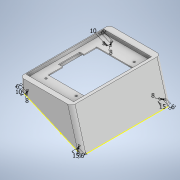
# Autodesk Inventor part: Front
Saved by Autodesk Inventor 2022 (Build 260153000, 153)
## iProperties
Created: 2021-06-27
Part Number: Front
Material: Generic
Document SubType Name: Modeling
Designer: Anton
Density: 1 g/cm^3
Appearance: Default
Author: Anton
Autodesk Inventor part; units mm, degrees
ref_plane "YZ Plane" through (0, 0, 0) normal (1, 0, 0) x (0, 1, 0)
ref_plane "XZ Plane" through (0, 0, 0) normal (0, 1, 0) x (-1, 0, 0)
ref_plane "XY Plane" through (0, 0, 0) normal (0, 0, 1) x (1, 0, 0)
sketch "Sketch1" plane through (0, 0, 0) normal (0, 1, 0) x (-1, 0, 0)
  line L0 (8, 0) -> (102.94, 0)
  line L1 (110.94, -8) -> (110.94, -185.2)
  line L2 (102.94, -193.2) -> (8, -193.2)
  line L3 (0, -185.2) -> (0, -8)
  circle A0 centre (86.7029, -32) radius 2.1
  circle A1 centre (88.297, -158.2) radius 2.1
  circle A2 centre (22.6, -158.501) radius 2.1
  circle A3 centre (21.4029, -32) radius 2.1
  arc A4 (110.94, -8) -> (102.94, 0) centre (102.94, -8) ccw
  arc A5 (8, 0) -> (0, -8) centre (8, -8) ccw
  arc A6 (0, -185.2) -> (8, -193.2) centre (8, -185.2) ccw
  arc A7 (102.94, -193.2) -> (110.94, -185.2) centre (102.94, -185.2) ccw
  point P0 (0, 0)
  dimension "d0" = 110.94
  dimension "d1" = 193.2
  dimension "d2" = 4.2
  dimension "d3" = 4.2
  dimension "d4" = 65.3
  dimension "d5" = 65.697
  dimension "d6" = 4.2
  dimension "d7" = 4.2
  dimension "d8" = 126.2
  dimension "d9" = 126.501
  dimension "d10" = 0
  dimension "d11" = 22.6
  dimension "d12" = 35
  dimension "d13" = 8
  constraints: 8 centre point, 8 end point, 8 point on circle, 8 tangent, 3 equal radius, 2 parallel, 2 point on line, 1 horizontal, 1 perpendicular
  measures "d0" distance between parallel lines of L3 L1
  measures "d1" distance between parallel lines of L2 L0
  measures "d2" diameter of A0
  measures "d3" diameter of A3
  measures "d4" distance of A3.centre A0.centre
  measures "d5" horizontal distance of A2.centre A1.centre
  measures "d6" diameter of A1
  measures "d7" diameter of A2
  measures "d8" vertical distance of A1.centre A0.centre
  measures "d9" vertical distance of A2.centre A3.centre
  measures "d10" vertical distance of A0.centre A3.centre
  measures "d11" distance from line of L3 A2.centre
  measures "d12" distance from line of L2 A1.centre
  measures "d13" radius of A4
extrude "Extrusion1" add sketch "Sketch1" along normal blind 2
sketch "Sketch2" plane through (0, 2, 0) normal (0, 1, 0) x (1, 0, 0)
  line L0 (-8, 193.2) -> (-102.94, 193.2) projected
  arc A0 (-102.94, 193.2) -> (-110.94, 185.2) centre (-102.94, 185.2) ccw projected
  line L1 (-110.94, 185.2) -> (-110.94, 8) projected
  arc A1 (-110.94, 8) -> (-102.94, 0) centre (-102.94, 8) ccw projected
  line L2 (-102.94, 0) -> (-8, 0) projected
  arc A2 (-8, 0) -> (0, 8) centre (-8, 8) ccw projected
  line L3 (0, 8) -> (0, 185.2) projected
  arc A3 (0, 185.2) -> (-8, 193.2) centre (-8, 185.2) ccw projected
  circle A4 centre (-86.7029, 32) radius 2.1 projected
  circle A5 centre (-88.297, 158.2) radius 2.1 projected
  circle A6 centre (-22.6, 158.501) radius 2.1 projected
  circle A7 centre (-21.4029, 32) radius 2.1 projected
  line L4 (-108.94, 11) -> (-108.94, 179.2)
  line L5 (-108.94, 179.2) -> (-6, 179.2)
  line L6 (-6, 11) -> (-108.94, 11)
  line L7 (-6, 179.2) -> (-6, 11)
  point P0 (0, 0)
  dimension "d16" = 2
  dimension "d17" = 14
  dimension "d18" = 11
  dimension "d19" = 6
  constraints: 8 end point, 1 horizontal
  measures "d16" distance between parallel lines of L1 L4
  measures "d17" distance between parallel lines of L0 L5
  measures "d18" distance between parallel lines of L2 L6
  measures "d19" distance between parallel lines of L3 L7
extrude "Extrusion2" add sketch "Sketch2" along normal blind 7.5 contours A3 L3 A2 L2 A1 L1 A0 L0
sketch "Sketch3" plane through (0, 2, 0) normal (0, 1, 0) x (1, 0, 0)
  line L0 (-91, 41) -> (-12, 41)
  line L1 (-12, 41) -> (-12, 146)
  line L2 (-12, 146) -> (-91, 146)
  line L3 (-6, 179.2) -> (-6, 11) projected
  line L4 (-6, 11) -> (-108.94, 11) projected
  line L5 (-99.94, 72) -> (-91, 72)
  line L6 (-91, 118.2) -> (-99.94, 118.2)
  line L7 (-99.94, 118.2) -> (-99.94, 72)
  circle A0 centre (-88.297, 158.2) radius 2.1 projected
  circle A1 centre (-86.7029, 32) radius 2.1 projected
  line L8 (-108.94, 11) -> (-108.94, 179.2) projected
  line L9 (-91, 146) -> (-91, 118.2)
  line L10 (-91, 72) -> (-91, 41)
  point P0 (0, 0)
  dimension "d22" = 105
  dimension "d24" = 6
  dimension "d25" = 30
  dimension "d26" = 40
  dimension "d27" = 40
  dimension "d28" = 9
  constraints: 16 end point, 4 parallel, 2 horizontal, 1 perpendicular
  measures "d22" distance between parallel lines of L2 L0
  measures "d24" distance between parallel lines of L3 L1
  measures "d25" distance between parallel lines of L4 L0
  measures "d26" distance from line of L6 A0.centre
  measures "d27" distance from line of L5 A1.centre
  measures "d28" distance between parallel lines of L8 L7
extrude "Extrusion3" cut sketch "Sketch3" against normal blind 7.5 contours L10 L5 L7 L6 L9 L2 L1 L0
sketch "Sketch5" plane through (0, 0, 0) normal (0, -1, 0) x (1, 0, 0)
  line L0 (-12, -146) -> (-91, -146) projected
  line L1 (-91, -146) -> (-91, -118.2) projected
  line L2 (-91, -118.2) -> (-99.94, -118.2) projected
  line L3 (-99.94, -118.2) -> (-99.94, -72) projected
  line L4 (-99.94, -72) -> (-91, -72) projected
  line L5 (-91, -72) -> (-91, -41) projected
  line L6 (-91, -41) -> (-12, -41) projected
  line L7 (-12, -41) -> (-12, -146) projected
  line L8 (-8, -193.2) -> (-102.94, -193.2) projected
  arc A0 (-8, -193.2) -> (0, -185.2) centre (-8, -185.2) ccw projected
  line L9 (0, -8) -> (0, -185.2) projected
  arc A1 (0, -8) -> (-8, 0) centre (-8, -8) ccw projected
  line L10 (-102.94, 0) -> (-8, 0) projected
  arc A2 (-102.94, 0) -> (-110.94, -8) centre (-102.94, -8) ccw projected
  line L11 (-110.94, -185.2) -> (-110.94, -8) projected
  arc A3 (-110.94, -185.2) -> (-102.94, -193.2) centre (-102.94, -185.2) ccw projected
  circle A4 centre (-86.7029, -32) radius 2.1 projected
  circle A5 centre (-88.297, -158.2) radius 2.1 projected
  circle A6 centre (-22.6, -158.501) radius 2.1 projected
  circle A7 centre (-21.4029, -32) radius 2.1 projected
  line L12 (-102.94, -191.2) -> (-8, -191.2)
  arc A8 (-8, -191.2) -> (-2, -185.2) centre (-8, -185.2) ccw
  line L13 (-2, -185.2) -> (-2, -8)
  arc A9 (-2, -8) -> (-8, -2) centre (-8, -8) ccw
  line L14 (-8, -2) -> (-102.94, -2)
  arc A10 (-102.94, -2) -> (-108.94, -8) centre (-102.94, -8) ccw
  line L15 (-108.94, -8) -> (-108.94, -185.2)
  arc A11 (-108.94, -185.2) -> (-102.94, -191.2) centre (-102.94, -185.2) ccw
  point P0 (0, 0)
  dimension "d39" = 2
  constraints: 8 end point, 8 point on circle, 4 centre point, 7 other
  measures "d39" radial gap between concentric circles of A3 A11
extrude "Extrusion4" add sketch "Sketch5" along normal blind 72 contours L8 A3 L11 A2 L10 A1 L9 A0
sketch "Sketch6" plane through (-8, 9.5, -193.2) normal (0, 0, -1) x (-1, 0, 0)
  line L0 (102.94, -81.5) -> (102.94, 0) projected
  line L1 (-8, -81.5) -> (102.94, -81.5)
  line L2 (102.94, -81.5) -> (102.94, -23.5)
  line L3 (102.94, 0) -> (94.94, 0) projected
  line L4 (-8, -81.5) -> (0, -81.5) projected
  line L5 (0, 0) -> (-8, 0) projected
  line L6 (0, 0) -> (94.94, 0) projected
  line L7 (102.94, -23.5) -> (-25.549, -79.0929)
  line L8 (-8, -81.5) -> (-29.8984, -81.5)
  line L9 (-29.8984, -81.5) -> (-31.1125, -81.5)
  line L10 (-25.549, -79.0929) -> (-31.1125, -81.5)
  line L11 (-8, -81.5) -> (-8, 0) projected
  point P0 (-8, -9.5)
  dimension "d42" = 23.5
  dimension "d47" = 23.396
  dimension "d48" = 140
  dimension "d51" = 23.1125
  constraints: 12 end point, 3 horizontal, 1 point on line
  measures "d42" distance from line of L3 L2.end
  measures "d47" angle of L6 L7
  measures "d48" distance of L2.end L7.end
  measures "d51" distance from line of L9.end L11
extrude "Extrusion5" cut sketch "Sketch6" along normal mid plane 1000 contours L1 L11 L7 L0 | L11 L8 L9 L10 L7
sketch "Sketch7" plane through (0, 9.5, 0) normal (0, 1, 0) x (1, 0, 0)
  arc A0 (-102.94, 193.2) -> (-110.94, 185.2) centre (-102.94, 185.2) ccw projected
  line L0 (-110.94, 185.2) -> (-110.94, 8) projected
  arc A1 (-110.94, 8) -> (-102.94, 0) centre (-102.94, 8) ccw projected
  line L1 (-102.94, 0) -> (-8, 0) projected
  arc A2 (-8, 0) -> (0, 8) centre (-8, 8) ccw projected
  line L2 (0, 8) -> (0, 185.2) projected
  arc A3 (0, 185.2) -> (-8, 193.2) centre (-8, 185.2) ccw projected
  line L3 (-8, 193.2) -> (-102.94, 193.2) projected
  line L4 (-108.94, 11) -> (-108.94, 179.2) projected
  line L5 (-108.94, 179.2) -> (-6, 179.2) projected
  line L6 (-6, 179.2) -> (-6, 11) projected
  line L7 (-6, 11) -> (-108.94, 11) projected
  line L8 (-8, 0) -> (23.113, 0)
  arc A4 (-8, 0) -> (0, 8) centre (-8, 8) ccw projected
  line L9 (23.113, 0) -> (23.113, 193.2)
  line L10 (23.113, 193.2) -> (-8, 193.2)
  arc A5 (0, 185.2) -> (-8, 193.2) centre (-8, 185.2) ccw projected
  point P0 (0, 0)
  point P1 (-8, 193.2)
  dimension "d52" = 23.113
  constraints: 6 end point, 2 perpendicular, 2 point on circle, 2 tangent, 1 horizontal
  measures "d52" distance between parallel lines of L2 L9
extrude "Extrusion6" add sketch "Sketch7" against normal up to surface contours L10 L9 L8 A2 L2 A3 surface through (-110.94, -14, -193.2) normal (0.397092, 0.9177788, 0)
sketch "Sketch8" plane through (-102.94, -17.4613, 0) normal (0, 0, 1) x (1, 0, 0)
  line L0 (126.053, 26.9613) -> (0, 26.9613) projected
  line L1 (126.053, 26.9613) -> (102.94, 26.9613)
  line L2 (0, 0) -> (126.053, -54.5389) projected
  line L3 (102.94, 26.9613) -> (126.053, -54.5389)
  line L4 (126.053, 26.9613) -> (126.053, -54.5389) projected
  line L5 (126.053, -54.5389) -> (126.053, 26.9613)
  point P0 (102.94, 17.4613)
  point P1 (96.94, 26.9613)
  dimension "d55" = 6
  constraints: 6 end point, 1 collinear, 1 point on line
  measures "d55" distance of point (96.94, 26.961) L1.end
extrude "Extrusion7" cut sketch "Sketch8" against normal blind 1000
sketch "Sketch9" plane through (0, 9.5, 0) normal (0, 1, 0) x (1, 0, 0)
  line L0 (23.113, 0) -> (0, 0) projected
  line L1 (-8, 0) -> (-110.94, 0)
  line L2 (-110.94, 0) -> (-110.94, 193.2)
  line L3 (-110.94, 193.2) -> (-8, 193.2)
  line L4 (0, 185.2) -> (0, 8)
  arc A0 (0, 185.2) -> (-8, 193.2) centre (-8, 185.2) ccw
  arc A1 (-8, 0) -> (0, 8) centre (-8, 8) ccw
  line L5 (0, 0) -> (0, 193.2) projected
  line L6 (0, 193.2) -> (0, 185.2)
  line L7 (-8, 193.2) -> (0, 193.2)
  line L8 (-102.94, 193.2) -> (23.113, 193.2) projected
  line L9 (-8, 0) -> (0, 0)
  line L10 (23.113, 0) -> (-102.94, 0) projected
  line L11 (0, 8) -> (0, 0)
  dimension "d58" = 8
  constraints: 16 end point, 6 tangent, 5 point on circle, 3 point on line, 2 centre point, 2 collinear, 2 parallel, 2 perpendicular, 1 equal radius, 1 horizontal
  measures "d58" radius of A0
sketch3d "3D Sketch1"
  line L0 (0, 9.5, 0) -> (23.113, -72.0002, 0)
sweep "Sweep1" cut profiles "Sketch9" path "3D Sketch1" contours A1 L5 L9 | A0 L7 L5
ref_plane "Work Plane1" through (23.113, -72.0002, -144.9) normal (-0.272835, 0.9620608, 0) x (0, 0, 1)
sketch "Sketch11" plane through (23.113, -72.0002, -144.9) normal (-0.272835, 0.9620608, 0) x (0, 0, 1)
  line L0 (-46.3, -106.3905) -> (-46.3, -26.2598) projected
  ellipse E0 centre (-40.3, -106.3905) end of major axis (-34.3, -106.3905) minor radius 5.0641 (-46.3, -106.3905) -> (-40.3, -111.4546) ccw projected
  line L1 (136.9, -111.4546) -> (-40.3, -111.4546) projected
  ellipse E1 centre (136.9, -106.3905) end of major axis (142.9, -106.3905) minor radius 5.0641 (136.9, -111.4546) -> (142.9, -106.3905) ccw projected
  line L2 (142.9, -26.2598) -> (142.9, -106.3905) projected
  ellipse E2 centre (136.9, -26.2598) end of major axis (130.9, -26.2598) minor radius 5.0641 (142.9, -26.2598) -> (136.9, -21.1957) ccw projected
  line L3 (-40.3, -21.1957) -> (136.9, -21.1957) projected
  ellipse E3 centre (-40.3, -26.2598) end of major axis (-46.3, -26.2598) minor radius 5.0641 (-40.3, -21.1957) -> (-46.3, -26.2598) ccw projected
  ellipse E4 centre (-40.3, -7.6965) end of major axis (-48.3, -7.6965) minor radius 7.6965 (-40.3, 0) -> (-48.3, -7.6965) ccw projected
  line L4 (-40.3, 0) -> (136.9, 0) projected
  ellipse E5 centre (136.9, -7.6965) end of major axis (144.9, -7.6965) minor radius 7.6965 (144.9, -7.6965) -> (136.9, 0) ccw projected
  line L5 (144.9, -7.6965) -> (144.9, -106.3905) projected
  ellipse E6 centre (136.9, -106.3905) end of major axis (144.9, -106.3905) minor radius 6.7521 (136.9, -113.1427) -> (144.9, -106.3905) ccw projected
  line L6 (-40.3, -113.1427) -> (136.9, -113.1427) projected
  ellipse E7 centre (-40.3, -106.3905) end of major axis (-32.3, -106.3905) minor radius 6.7521 (-48.3, -106.3905) -> (-40.3, -113.1427) ccw projected
  line L7 (-48.3, -106.3905) -> (-48.3, -7.6965) projected
  line L8 (142.9, -106.3905) -> (142.9, -7.6965)
  line L9 (136.9, -2) -> (-40.3, -2)
  line L10 (-46.3, -7.6965) -> (-46.3, -106.3905)
  line L11 (-40.3, -111.1427) -> (136.9, -111.1427)
  spline S0 degree 5 poles (142.9, -7.6965) (142.9001, -6.8006) (142.7143, -5.9048) (142.3427, -5.0609) (141.2621, -3.5342) (139.6817, -2.5262) (138.7833, -2.1755) (137.8416, -2.0001) (136.9, -2) knots 0 0 0 0 0 0 0.487536 0.487536 0.487536 1 1 1 1 1 1
  spline S1 degree 5 poles (-40.3, -2) (-41.2416, -2.0001) (-42.1833, -2.1755) (-43.0817, -2.5262) (-44.6621, -3.5342) (-45.7427, -5.0609) (-46.1143, -5.9048) (-46.3001, -6.8006) (-46.3, -7.6965) knots 0 0 0 0 0 0 0.512464 0.512464 0.512464 1 1 1 1 1 1
  spline S2 degree 5 poles (-46.3, -106.3905) (-46.3, -106.7934) (-46.245, -107.1962) (-46.1354, -107.5891) (-45.6891, -108.6469) (-44.9171, -109.5209) (-44.3279, -109.9845) (-43.1975, -110.6308) (-41.951, -110.9896) (-41.4049, -111.0916) (-40.8524, -111.1427) (-40.3, -111.1427) knots 0 0 0 0 0 0 0.23796 0.23796 0.23796 0.673702 0.673702 0.673702 1 1 1 1 1 1
  spline S3 degree 5 poles (136.9, -111.1427) (137.4524, -111.1427) (138.0049, -111.0916) (138.551, -110.9896) (139.7975, -110.6308) (140.9279, -109.9845) (141.5171, -109.5209) (142.2891, -108.6469) (142.7354, -107.5891) (142.845, -107.1962) (142.9, -106.7934) (142.9, -106.3905) knots 0 0 0 0 0 0 0.326298 0.326298 0.326298 0.76204 0.76204 0.76204 1 1 1 1 1 1
  point P0 (-46.3, -26.2598)
  dimension "d64" = 2
  constraints: 8 end point, 7 parallel, 20 other
  measures "d64" distance between parallel lines of L5 L8
extrude "Extrusion8" cut sketch "Sketch11" along normal up to surface contours L10 S1 L9 S0 L8 E2 L3 E3 surface through (-55.47, 0, -96.6) normal (0, 1, 0)
sketch "Sketch12" plane through (-110.94, -14, -185.2) normal (-0.397092, -0.9177788, 0) x (0.9177788, -0.397092, 0)
  circle A0 centre (10, 179.2) radius 4
  circle A1 centre (131.0624, 179.2) radius 4
  circle A2 centre (10, -2) radius 4
  circle A3 centre (131.0624, -2) radius 4
  line L0 (146.0624, 0) -> (146.0624, 177.2) projected
  line L1 (136.1266, 185.2) -> (8.7167, 185.2) projected
  line L2 (8.7167, -8) -> (136.1266, -8) projected
  line L3 (0, 0) -> (0, 177.2) projected
  point P0 (96.2591, 185.2)
  dimension "d67" = 8
  dimension "d68" = 8
  dimension "d69" = 8
  dimension "d70" = 8
  dimension "d71" = 15
  dimension "d72" = 6
  dimension "d73" = 6
  dimension "d74" = 15
  dimension "d75" = 6
  dimension "d76" = 10
  dimension "d77" = 6
  dimension "d78" = 10
  constraints: 4 centre point
  measures "d67" diameter of A2
  measures "d68" diameter of A3
  measures "d69" diameter of A1
  measures "d70" diameter of A0
  measures "d71" distance from line of L0 A1.centre
  measures "d72" distance from line of L1 A1.centre
  measures "d73" distance from line of L2 A3.centre
  measures "d74" distance from line of L0 A3.centre
  measures "d75" distance from line of L1 A0.centre
  measures "d76" distance from line of L3 A0.centre
  measures "d77" distance from line of L2 A2.centre
  measures "d78" distance from line of L3 A2.centre
sketch "Sketch13" plane through (-110.94, -14, -185.2) normal (-0.397092, -0.9177788, 0) x (0.9177788, -0.397092, 0)
  line L0 (8.7167, -6) -> (136.1266, -6) projected
  ellipse E0 centre (8.7167, 0) end of major axis (15.2542, 0) minor radius 6 (2.1792, 0) -> (8.7167, -6) ccw projected
  line L1 (2.1792, 177.2) -> (2.1792, 0) projected
  ellipse E1 centre (8.7167, 177.2) end of major axis (15.2542, 177.2) minor radius 6 (8.7167, 183.2) -> (2.1792, 177.2) ccw projected
  line L2 (136.1266, 183.2) -> (8.7167, 183.2) projected
  spline S0 degree 7 poles (136.1266, 183.2) (136.5145, 183.2) (136.9024, 183.1805) (137.2895, 183.1415) (137.6749, 183.0829) (138.0577, 183.0043) (138.4369, 182.9054) (139.1571, 182.6749) (139.4987, 182.5464) (139.8353, 182.3995) (140.1657, 182.2338) (140.4886, 182.0484) (140.8022, 181.8427) (141.2991, 181.4697) (141.4891, 181.3148) (141.6737, 181.151) (141.8524, 180.978) (142.0243, 180.7958) (142.1886, 180.6042) (142.4577, 180.2566) (142.5665, 180.1051) (142.6703, 179.9487) (142.7687, 179.7873) (142.8612, 179.6212) (142.9472, 179.4504) (143.1497, 179.0025) (143.2564, 178.7189) (143.3444, 178.4258) (143.412, 178.1251) (143.4577, 177.8187) (143.4805, 177.5093) (143.4805, 177.2) knots 0 0 0 0 0 0 0 0 0.275632 0.275632 0.275632 0.275632 0.275632 0.275632 0.530207 0.530207 0.530207 0.530207 0.530207 0.530207 0.694174 0.694174 0.694174 0.694174 0.694174 0.694174 0.813721 0.813721 0.813721 0.813721 0.813721 0.813721 1 1 1 1 1 1 1 1 projected
  line L3 (143.4805, 177.2) -> (143.4805, 0) projected
  spline S1 degree 7 poles (143.4805, 0) (143.4805, -0.3097) (143.4576, -0.6195) (143.4118, -0.9263) (143.3441, -1.2275) (143.2558, -1.5208) (143.1489, -1.8047) (142.9457, -2.2535) (142.8593, -2.4247) (142.7664, -2.5913) (142.6676, -2.7531) (142.5633, -2.9099) (142.454, -3.0618) (142.1848, -3.4086) (142.021, -3.5993) (141.8496, -3.7807) (141.6715, -3.9529) (141.4875, -4.116) (141.2983, -4.2703) (140.8031, -4.642) (140.4906, -4.847) (140.1689, -5.0319) (139.8397, -5.1973) (139.5043, -5.3439) (139.164, -5.4723) (138.444, -5.7036) (138.0637, -5.8031) (137.6797, -5.8822) (137.2931, -5.9412) (136.9048, -5.9804) (136.5157, -6) (136.1266, -6) knots 0 0 0 0 0 0 0 0 0.186527 0.186527 0.186527 0.186527 0.186527 0.186527 0.306463 0.306463 0.306463 0.306463 0.306463 0.306463 0.469804 0.469804 0.469804 0.469804 0.469804 0.469804 0.72351 0.72351 0.72351 0.72351 0.72351 0.72351 1 1 1 1 1 1 1 1 projected
  ellipse E2 centre (136.1266, 0) end of major axis (126.1907, 0) minor radius 8 (136.1266, -8) -> (146.0624, 0) ccw projected
  line L4 (146.0624, 0) -> (146.0624, 177.2) projected
  ellipse E3 centre (136.1266, 177.2) end of major axis (146.0624, 177.2) minor radius 8 (146.0624, 177.2) -> (136.1266, 185.2) ccw projected
  line L5 (136.1266, 185.2) -> (8.7167, 185.2) projected
  ellipse E4 centre (8.7167, 177.2) end of major axis (0, 177.2) minor radius 8 (8.7167, 185.2) -> (0, 177.2) ccw projected
  line L6 (0, 0) -> (0, 177.2) projected
  ellipse E5 centre (8.7167, 0) end of major axis (0, 0) minor radius 8 (0, 0) -> (8.7167, -8) ccw projected
  line L7 (8.7167, -8) -> (136.1266, -8) projected
  line L8 (91.3895, 183.2) -> (1.7829, 183.2) projected
  line L9 (15.1792, 175.2) -> (2.1792, 175.2)
  line L10 (2.1792, 177.2) -> (2.1792, 0) projected
  line L11 (15.1792, 183.2) -> (15.1792, 175.2)
  line L12 (-4.5179, 174.2) -> (89.9582, 174.2) projected
  line L13 (1.7829, -6) -> (91.3895, -6) projected
  line L14 (15.1792, -6) -> (15.1792, 2)
  line L15 (15.1792, 2) -> (2.1792, 2)
  line L16 (143.4805, 177.2) -> (143.4805, 0) projected
  line L17 (143.4805, 2) -> (126.4805, 2)
  line L18 (126.4805, 2) -> (126.4805, -6)
  line L19 (136.1266, -6) -> (91.3895, -6) projected
  line L20 (136.1266, 183.2) -> (91.3895, 183.2) projected
  line L21 (126.4805, 183.2) -> (126.4805, 175.2)
  line L22 (126.4805, 175.2) -> (143.4805, 175.2)
  point P0 (96.2591, 185.2)
  point P1 (143.4805, 2)
  point P2 (126.4805, -6)
  dimension "d80" = 13
  dimension "d81" = 8
  dimension "d82" = 8
  dimension "d83" = 13
  dimension "d84" = 17
  dimension "d85" = 8
  dimension "d86" = 8
  dimension "d87" = 17
  constraints: 16 end point, 8 point on line, 7 perpendicular, 8 other
  measures "d80" distance of L9.start L9.end
  measures "d81" distance of L11.start L9.start
  measures "d82" distance of L14.start L14.end
  measures "d83" distance of L14.end L15.end
  measures "d84" distance of L17.start L17.end
  measures "d85" distance of L17.end L18.end
  measures "d86" distance of L21.start L21.end
  measures "d87" distance of L21.end L22.end
sketch3d "3D Sketch2"
  line L0 (20.7434, -70.975, -185.2) -> (0.6153, 0, -185.2)
sweep "Sweep2" add profiles "Sketch13" path "3D Sketch2" contours L18 L17 L3 S1 L0 | L22 L21 L2 S0 L3
sketch "Sketch14" plane through (-110.94, -14, -185.2) normal (-0.397092, -0.9177788, 0) x (0.9177788, -0.397092, 0)
  line L0 (8.7167, -6) -> (126.4805, -6) projected
  ellipse E0 centre (8.7167, 0) end of major axis (15.2542, 0) minor radius 6 (2.1792, 0) -> (8.7167, -6) ccw projected
  line L1 (2.1792, 177.2) -> (2.1792, 0) projected
  ellipse E1 centre (8.7167, 177.2) end of major axis (15.2542, 177.2) minor radius 6 (8.7167, 183.2) -> (2.1792, 177.2) ccw projected
  line L2 (126.4805, 183.2) -> (8.7167, 183.2) projected
  line L3 (126.4805, 183.2) -> (126.4805, 175.2) projected
  line L4 (126.4805, 175.2) -> (143.4805, 175.2) projected
  line L5 (143.4805, 175.2) -> (143.4805, 2) projected
  line L6 (143.4805, 2) -> (126.4805, 2) projected
  line L7 (126.4805, 2) -> (126.4805, -6) projected
  ellipse E2 centre (136.1266, 0) end of major axis (126.1907, 0) minor radius 8 (136.1266, -8) -> (146.0624, 0) ccw projected
  line L8 (146.0624, 0) -> (146.0624, 177.2) projected
  ellipse E3 centre (136.1266, 177.2) end of major axis (146.0624, 177.2) minor radius 8 (146.0624, 177.2) -> (136.1266, 185.2) ccw projected
  line L9 (136.1266, 185.2) -> (8.7167, 185.2) projected
  ellipse E4 centre (8.7167, 177.2) end of major axis (0, 177.2) minor radius 8 (8.7167, 185.2) -> (0, 177.2) ccw projected
  line L10 (0, 0) -> (0, 177.2) projected
  ellipse E5 centre (8.7167, 0) end of major axis (0, 0) minor radius 8 (0, 0) -> (8.7167, -8) ccw projected
  line L11 (8.7167, -8) -> (136.1266, -8) projected
  line L12 (8.7167, -6) -> (126.4805, -6) projected
  line L13 (15.1792, -6) -> (15.1792, 2)
  line L14 (15.1792, 2) -> (2.1792, 2)
  line L15 (84.2614, 183.2) -> (1.7829, 183.2) projected
  line L16 (15.1792, 183.2) -> (15.1792, 175.2)
  line L17 (15.1792, 175.2) -> (2.1792, 175.2)
  line L18 (2.1792, 177.2) -> (2.1792, 0) projected
  point P0 (96.2591, 185.2)
  point P1 (15.1792, -6)
  point P2 (15.1792, 183.2)
  dimension "d90" = 13
  dimension "d91" = 8
  dimension "d92" = 13
  dimension "d93" = 8
  constraints: 8 end point, 4 point on line, 2 perpendicular, 2 vertical, 6 other
  measures "d90" distance of L13.end L14.end
  measures "d91" distance of L13.start L13.end
  measures "d92" distance of L16.end L17.end
  measures "d93" distance of L16.start L16.end
sketch3d "3D Sketch3"
  line L0 (-102.94, -17.4613, -191.2) -> (-102.94, 0, -191.2)
sweep "Sweep3" add profiles "Sketch14" path "3D Sketch3" contours E0 L1 L14 L13 L0 | L1 E1 L2 L16 L17
body "Solid1"
